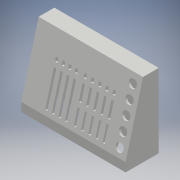
# Autodesk Inventor part: SoundBoard
Saved by Autodesk Inventor 2018 (Build 220112000, 112)
## iProperties
Created: 2017-09-09
Part Number: SoundBoard
Material: Generic
Document SubType Name: Modeling
Designer: Ahmed Alhag
Density: 1 g/cm^3
Appearance: Default
Author: Ahmed Alhag
Autodesk Inventor part; units mm, degrees
ref_plane "YZ Plane" through (0, 0, 0) normal (1, 0, 0) x (0, 1, 0)
ref_plane "XZ Plane" through (0, 0, 0) normal (0, 1, 0) x (-1, 0, 0)
ref_plane "XY Plane" through (0, 0, 0) normal (0, 0, 1) x (1, 0, 0)
sketch "Sketch5" plane through (0, 0, 0) normal (1, 0, 0) x (0, 1, 0)
  line L0 (0, -90.3407) -> (198.8643, -90.3407)
  line L1 (198.8643, -90.3407) -> (198.8643, -42.9328)
  line L2 (198.8643, -42.9328) -> (2.5882, 9.6593)
  line L3 (-24, 9.6593) -> (-24, -90.3407)
  line L4 (-24, -90.3407) -> (0, -90.3407)
  line L5 (2.5882, 9.6593) -> (198.8643, -42.9328)
  line L6 (2.5882, 9.6593) -> (-24, 9.6593)
  point P0 (0, 0)
  point P1 (0, 0)
  dimension "d214" = 100
  dimension "d216" = 24
  dimension "d218" = 15
  dimension "d219" = 47.408
  constraints: 14 end point, 2 perpendicular, 1 collinear, 1 point on line
  measures "d214" distance of L3.start L3.end
  measures "d216" distance of L0.start L3.end
  measures "d218" angle of L2 L6
  measures "d219" distance of L0.end L1.end
extrude "Extrusion5" add sketch "Sketch5" along normal mid plane 314.96
shell "Shell1" thickness 7 removed faces 1 at (-52.4933, -24, -23.6741)
sketch "Sketch6" plane through (-157.48, 2.5882, 9.6593) normal (0, 0.2588, 0.9659) x (1, 0, 0)
  line L0 (314.96, -3.925) -> (314.96, 199.275)
  line L1 (0, 0) -> (314.96, 0)
  line L2 (314.96, 0) -> (314.96, 199.275)
  circle A0 centre (290.96, 24) radius 12
  line L3 (135.21, 13) -> (135.21, 114.75)
  line L4 (69.21, 114.75) -> (69.21, 13)
  line L5 (128.46, 114.75) -> (128.46, 13)
  line L6 (108.71, 114.75) -> (108.71, 13)
  line L7 (88.96, 114.75) -> (88.96, 13)
  line L8 (115.46, 13) -> (115.46, 114.75)
  line L9 (95.71, 13) -> (95.71, 114.75)
  line L10 (75.96, 13) -> (75.96, 114.75)
  line L11 (135.21, 114.75) -> (128.46, 114.75)
  line L12 (115.46, 114.75) -> (108.71, 114.75)
  line L13 (95.71, 114.75) -> (88.96, 114.75)
  line L14 (75.96, 114.75) -> (69.21, 114.75)
  line L15 (248.96, 71) -> (242.21, 71)
  line L16 (242.21, 71) -> (242.21, 116)
  line L17 (227.21, 116) -> (227.21, 71)
  line L18 (227.21, 71) -> (220.46, 71)
  line L19 (220.46, 71) -> (220.46, 116)
  line L20 (248.96, 116) -> (248.96, 71)
  line L21 (69.21, 13) -> (75.96, 13)
  line L22 (88.96, 13) -> (95.71, 13)
  line L23 (108.71, 13) -> (115.46, 13)
  line L24 (128.46, 13) -> (135.21, 13)
  line L25 (183.71, 71) -> (176.96, 71)
  line L26 (205.46, 71) -> (198.71, 71)
  line L27 (183.71, 116) -> (183.71, 71)
  line L28 (198.71, 71) -> (198.71, 116)
  line L29 (205.46, 116) -> (205.46, 71)
  line L30 (176.96, 71) -> (176.96, 116)
  line L31 (220.4664, 58) -> (227.2164, 58)
  line L32 (227.2164, 58) -> (227.2164, 13)
  line L33 (227.2164, 13) -> (220.4664, 13)
  line L34 (242.2164, 58) -> (248.9664, 58)
  line L35 (242.2164, 13) -> (242.2164, 58)
  line L36 (248.9664, 13) -> (242.2164, 13)
  line L37 (248.9664, 58) -> (248.9664, 13)
  line L38 (220.4664, 13) -> (220.4664, 58)
  line L39 (155.21, 13) -> (155.21, 58)
  line L40 (155.21, 58) -> (161.9664, 58)
  line L41 (161.9664, 58) -> (161.9664, 13)
  line L42 (205.4664, 58) -> (205.4664, 13)
  line L43 (198.7164, 58) -> (205.4664, 58)
  line L44 (198.7164, 13) -> (198.7164, 58)
  line L45 (205.4664, 13) -> (198.7164, 13)
  line L46 (183.7164, 58) -> (183.7164, 13)
  line L47 (176.9664, 13) -> (176.9664, 58)
  line L48 (183.7164, 13) -> (176.9664, 13)
  line L49 (161.9664, 13) -> (155.21, 13)
  line L50 (176.9664, 58) -> (183.7164, 58)
  line L51 (155.21, 71) -> (155.21, 116)
  line L52 (161.96, 71) -> (155.21, 71)
  line L53 (161.96, 116) -> (161.96, 71)
  line L54 (155.21, 116) -> (161.96, 116)
  line L55 (76.585, 127.75) -> (76.585, 139.75)
  line L56 (76.585, 139.75) -> (68.585, 139.75)
  line L57 (68.585, 139.75) -> (68.585, 127.75)
  line L58 (68.585, 127.75) -> (76.585, 127.75)
  line L59 (176.96, 116) -> (183.71, 116)
  line L60 (198.71, 116) -> (205.46, 116)
  line L61 (220.46, 116) -> (227.21, 116)
  line L62 (242.21, 116) -> (248.96, 116)
  circle A1 centre (290.96, 62) radius 12
  circle A2 centre (290.96, 100) radius 12
  circle A3 centre (290.96, 138) radius 12
  circle A4 centre (290.96, 176) radius 12
  line L63 (96.285, 139.75) -> (88.285, 139.75)
  line L64 (96.285, 127.75) -> (96.285, 139.75)
  line L65 (88.285, 127.75) -> (96.285, 127.75)
  line L66 (88.285, 139.75) -> (88.285, 127.75)
  line L67 (115.985, 139.75) -> (107.985, 139.75)
  line L68 (115.985, 127.75) -> (115.985, 139.75)
  line L69 (107.985, 127.75) -> (115.985, 127.75)
  line L70 (107.985, 139.75) -> (107.985, 127.75)
  line L71 (135.685, 139.75) -> (127.685, 139.75)
  line L72 (135.685, 127.75) -> (135.685, 139.75)
  line L73 (127.685, 127.75) -> (135.685, 127.75)
  line L74 (127.685, 139.75) -> (127.685, 127.75)
  line L75 (154.585, 127.75) -> (162.585, 127.75)
  line L76 (162.585, 127.75) -> (162.585, 139.75)
  line L77 (162.585, 139.75) -> (154.585, 139.75)
  line L78 (154.585, 139.75) -> (154.585, 127.75)
  line L79 (176.335, 139.75) -> (176.335, 127.75)
  line L80 (184.335, 139.75) -> (176.335, 139.75)
  line L81 (184.335, 127.75) -> (184.335, 139.75)
  line L82 (176.335, 127.75) -> (184.335, 127.75)
  line L83 (198.085, 139.75) -> (198.085, 127.75)
  line L84 (206.085, 139.75) -> (198.085, 139.75)
  line L85 (206.085, 127.75) -> (206.085, 139.75)
  line L86 (198.085, 127.75) -> (206.085, 127.75)
  line L87 (219.835, 139.75) -> (219.835, 127.75)
  line L88 (227.835, 139.75) -> (219.835, 139.75)
  line L89 (227.835, 127.75) -> (227.835, 139.75)
  line L90 (219.835, 127.75) -> (227.835, 127.75)
  line L91 (241.585, 139.75) -> (241.585, 127.75)
  line L92 (249.585, 139.75) -> (241.585, 139.75)
  line L93 (249.585, 127.75) -> (249.585, 139.75)
  line L94 (241.585, 127.75) -> (249.585, 127.75)
  line L95 (0, 0) -> (314.96, 0) projected
  line L96 (0, 203.2) -> (314.96, 203.2) projected
  line L97 (314.96, 203.2) -> (314.96, 0) projected
  dimension "d226" = 314.96
  dimension "d232" = 101.75
  dimension "d233" = 6.75
  dimension "d234" = 45
  dimension "d235" = 6.7564
  dimension "d236" = 13
  dimension "d237" = 13
  dimension "d238" = 13
  dimension "d239" = 6.75
  dimension "d240" = 6.75
  dimension "d241" = 6.75
  dimension "d242" = 101.75
  dimension "d243" = 101.75
  dimension "d244" = 101.75
  dimension "d245" = 0
  dimension "d246" = 0
  dimension "d247" = 0
  dimension "d253" = 13
  dimension "d254" = 13
  dimension "d255" = 45
  dimension "d256" = 45
  dimension "d257" = 45
  dimension "d258" = 45
  dimension "d259" = 13
  dimension "d260" = 13
  dimension "d261" = 13
  dimension "d262" = 6.75
  dimension "d263" = 6.75
  dimension "d264" = 6.75
  dimension "d265" = 6.75
  dimension "d266" = 6.75
  dimension "d267" = 45
  dimension "d268" = 45
  dimension "d269" = 45
  dimension "d270" = 45
  dimension "d271" = 45
  dimension "d272" = 15
  dimension "d273" = 15
  dimension "d274" = 15
  dimension "d275" = 15
  dimension "d276" = 6.75
  dimension "d277" = 6.75
  dimension "d278" = 6.75
  dimension "d279" = 6.75
  dimension "d281" = 15
  dimension "d290" = 15
  dimension "d291" = 15
  dimension "d292" = 15
  dimension "d315" = 24
  dimension "d316" = 24
  dimension "d317" = 24
  dimension "d318" = 203.2
  dimension "d321" = 38
  dimension "SW" = 8
  dimension "SL" = 12
  dimension "d330" = 0.625
  dimension "d333" = 19.7
  dimension "d346" = 8
  dimension "d347" = 12
  dimension "d348" = 0.625
  dimension "d351" = 21.75
  dimension "d356" = 13
  dimension "d357" = 13
  dimension "d358" = 0
  constraints: 190 end point, 9 perpendicular, 5 centre point, 2 horizontal, 1 vertical, 64 other
  measures "d226" distance of L1.end L1.start
  measures "d232" distance of L14.end L4.end
  measures "d233" distance between parallel lines of L10 L4
  measures "d234" distance of L40.end L41.end
  measures "d235" distance of L40.start L40.end
  measures "d236" distance between parallel lines of L5 L8
  measures "d237" distance between parallel lines of L7 L10
  measures "d238" distance between parallel lines of L6 L9
  measures "d239" distance between parallel lines of L9 L7
  measures "d240" distance between parallel lines of L8 L6
  measures "d241" distance between parallel lines of L3 L5
  measures "d242" distance of L13.end L7.end
  measures "d243" distance of L12.end L6.end
  measures "d244" distance of L11.end L5.end
  measures "d245" distance between parallel lines of L12 L11
  measures "d246" distance between parallel lines of L13 L12
  measures "d247" distance between parallel lines of L14 L13
  measures "d253" distance between parallel lines of L52 L40
  measures "d254" distance between parallel lines of L25 L50
  measures "d255" distance of L48.end L50.start
  measures "d256" distance of L43.end L42.end
  measures "d257" distance of L33.end L31.start
  measures "d258" distance of L35.start L34.start
  measures "d259" distance between parallel lines of L26 L43
  measures "d260" distance between parallel lines of L31 L18
  measures "d261" distance between parallel lines of L34 L15
  measures "d262" distance of L54.start L53.start
  measures "d263" distance between parallel lines of L27 L30
  measures "d264" distance between parallel lines of L29 L28
  measures "d265" distance between parallel lines of L17 L19
  measures "d266" distance between parallel lines of L20 L16
  measures "d267" distance between parallel lines of L54 L52
  measures "d268" distance of L30.end L25.end
  measures "d269" distance of L29.start L29.end
  measures "d270" distance of L19.end L19.start
  measures "d271" distance of L16.end L16.start
  measures "d272" distance between parallel lines of L30 L53
  measures "d273" distance between parallel lines of L28 L27
  measures "d274" distance between parallel lines of L19 L29
  measures "d275" distance between parallel lines of L16 L17
  measures "d276" distance between parallel lines of L46 L47
  measures "d277" distance between parallel lines of L42 L44
  measures "d278" distance between parallel lines of L32 L38
  measures "d279" distance between parallel lines of L37 L35
  measures "d281" distance between parallel lines of L47 L41
  measures "d290" distance between parallel lines of L44 L46
  measures "d291" distance between parallel lines of L42 L38
  measures "d292" distance between parallel lines of L35 L32
  measures "d315" diameter of A0
  measures "d316" distance from line of L1 A0.centre
  measures "d317" distance from line of L0 A0.centre
  measures "d318" distance of L0.start L0.end
  measures "d321" distance of A0.centre A1.centre
  measures "SW" distance between parallel lines of L55 L57
  measures "SL" distance of L56.end L58.start
  measures "d330" distance between parallel lines of L4 L57
  measures "d333" distance of L56.end L63.end
  measures "d346" distance between parallel lines of L76 L78
  measures "d347" distance of L77.end L75.start
  measures "d348" distance between parallel lines of L78 L51
  measures "d351" distance of L77.end L79.start
  measures "d356" distance between parallel lines of L14 L58
  measures "d357" distance between parallel lines of L1 L21
  measures "d358" distance between parallel lines of L95 L1
extrude "Extrusion8" cut sketch "Sketch6" against normal up to next
body "Solid2"
body "Solid3"
